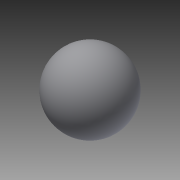
# Autodesk Inventor part: WBC6-12ZZ Ball
Saved by Autodesk Inventor 2014 SP2 (Build 180246200, 246)
## iProperties
Created: 2019-09-21
Part Number: WBC6-12ZZ Ball
Material: Generic
Catalog Web Link: www.cadenas.de
Description: Six types ball-Metric system sizes
Vendor: NTN
Document SubType Name: Modeling
Designer: psadmin
Manufacturer: NTN
Mass: 0.0029331 g
Surface Area: 0.0990914 cm^2
Volume: 0.0029331 cm^3
Density: 1 g/cm^3
Appearance: PSOLRGB-192-192-192
Category: PARTsolutions
Company: NTN
Title: WBC6-12ZZ Ball
Author: Cadenas PARTsolutions
Comments: Metric system sizes
PSOL_IDENT_0: {$CADENAS_DATA\23d-libs\ntn\ball_roller_bearings\miniature_extra_small_bb\metric_system_sizes\mss_ba
PSOL_IDENT_1: ll.prj},179 {VTYP=3D},{NB=WBC6-12ZZ Ball},{LINA=WBC6-12ZZ Ball},{NN=Six types ball},{DATE=29.01.2019
PSOL_IDENT_2: 23:03:32},{GEOMDATE=02.04.2007 00:00:00},{VERSION=},{LINEID=12850},{WBVAR=},{WBNUMERIC=}  {NB=WBC6-
PSOL_IDENT_3: 12ZZ Ball},{LINA=WBC6-12ZZ Ball},{KT=DUMMY},{IDNR=},{SD=6.0},{D=12},{B=3.0},{R=0.15},{ORDER=WBC6-12Z
PSOL_IDENT_4: Z},{CR=830},{COR=365},{CRF=85},{CORF=37},{LSG=40 000},{LSO=47 000},{MASS=1.30},{ORDER1=BC6-12},{D1=1
PSOL_IDENT_5: 3.2},{D2=13.6},{C1=0.6},{C2=0.8},{WSS=WBC6-12ZZ},{WDS=ZZ},{UTWF=FLBC6-12},{FORSS=FLAWBC6-12Z},{FORDS=
PSOL_IDENT_6: ZZ},{DA1=7,2},{DA2=7,9},{DA=10,8},{RAS=0,15},{MASS1=1.40},{B1=4.0},{VERS=3},{X=3},{N=9},{O=28.26},{R
PSOL_IDENT_7: B=0.888}
NN: Six types ball
NT: Metric system sizes
NB: WBC6-12ZZ Ball
NBSYN: $ORDER. Ball
LINA: WBC6-12ZZ Ball
SD: 6
D: 12
B: 3
R: 0.15
CR: 830
COR: 365
CRF: 85
CORF: 37
LSG: 40 000
LSO: 47 000
MASS: 1.3
ORDER1: BC6-12
D1: 13.2
D2: 13.6
C1: 0.6
C2: 0.8
WSS: WBC6-12ZZ
WDS: ZZ
UTWF: FLBC6-12
FORSS: FLAWBC6-12Z
FORDS: ZZ
DA1: 7,2
DA2: 7,9
DA: 10,8
RAS: 0,15
MASS1: 1.4
B1: 4
VERS: 3
SUPPLIER: NTN
ARTICLENO: WBC6-12ZZ Ball
BOMINFO: WBC6-12ZZ Ball
CREATOR: CADENAS GmbH
Autodesk Inventor part; units mm, degrees
sketch "Sketch_1" plane through (0, 0, 0) normal (0, 0, 1) x (1, 0, 0)
  line L0 (0.888, 0) -> (-0.888, 0)
  arc A0 (0.888, 0) -> (-0.888, 0) centre (0, 0) ccw
  line L1 (0.888, 0) -> (-0.888, 0)
  constraints: 4 end point, 2 point on circle, 1 centre point
revolve "Revolution1" add sketch "Sketch_1" angle 360 about axis through (0.888, 0, 0) along (1, 0, 0)
ref_plane "mss_ball_XY" through (0, 0, 0) normal (1, 0, 0) x (0, 0, -1)
ref_plane "mss_ball_YZ" through (0, 0, 0) normal (0, 0, -1) x (0, 1, 0)
ref_plane "mss_ball_ZX" through (0, 0, 0) normal (0, 1, 0) x (1, 0, 0)
body "Solid1"
